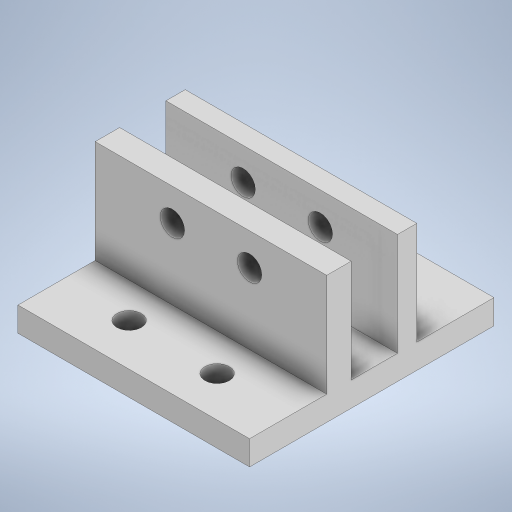
# Autodesk Inventor part: arm_to_tower_adapter
Saved by Autodesk Inventor 2024 (Build 280153000, 153)
## iProperties
Created: 2023-11-02
Part Number: arm_to_tower_adapter
Material: Generic
Document SubType Name: Modeling
Designer: dimademler
Density: 1 g/cm^3
Appearance: Default
Author: dimademler
Autodesk Inventor part; units mm, degrees
ref_plane "YZ Plane" through (0, 0, 0) normal (1, 0, 0) x (0, 1, 0)
ref_plane "XZ Plane" through (0, 0, 0) normal (0, 1, 0) x (-1, 0, 0)
ref_plane "XY Plane" through (0, 0, 0) normal (0, 0, 1) x (1, 0, 0)
sketch "Sketch1" plane through (0, 0, 0) normal (0, 0, 1) x (1, 0, 0)
  line L0 (0, 0) -> (-45.72, 0)
  line L1 (-45.72, 0) -> (-45.72, 20.32)
  line L2 (-45.72, 20.32) -> (0, 20.32)
  line L3 (0, 20.32) -> (0, 0)
  dimension "d0" = 45.72
  dimension "d1" = 20.32
  constraints: 8 end point, 2 parallel, 1 horizontal, 1 perpendicular
  measures "d0" distance of L0.start L0.end
  measures "d1" distance of L0.end L1.end
extrude "Extrusion1" add sketch "Sketch1" along normal blind 4.826
sketch "Sketch2" plane through (-45.72, 0, 0) normal (0, -1, 0) x (1, 0, 0)
  line L0 (45.72, 0) -> (45.72, 4.826) projected
  line L1 (0, 0) -> (0, 4.826) projected
  line L2 (0, 0) -> (45.72, 0) projected
  line L3 (0, 4.826) -> (45.72, 4.826) projected
  line L4 (45.72, 0) -> (45.72, -28.194)
  line L5 (45.72, 4.826) -> (45.72, 20.066)
  line L6 (45.72, 20.066) -> (0, 20.066)
  line L7 (0, 20.066) -> (0, 4.826)
  line L8 (0, 0) -> (0, -28.194)
  line L9 (0, -28.194) -> (45.72, -28.194)
  line L10 (45.72, 0) -> (45.72, 4.826)
  line L11 (0, 4.826) -> (0, 0)
  dimension "d4" = 28.194
  dimension "d5" = 15.24
  constraints: 16 end point, 4 vertical, 3 perpendicular, 1 point on line
  measures "d4" distance of L0.start L4.end
  measures "d5" distance of L0.end L5.end
extrude "Extrusion2" add sketch "Sketch2" along normal blind 4.826
sketch "Sketch3" plane through (-45.72, 0, 0) normal (0, 1, 0) x (1, 0, 0)
  line L0 (45.72, 0) -> (0, 0) projected
  line L1 (45.72, 28.194) -> (45.72, 0) projected
  line L2 (0, 28.194) -> (45.72, 28.194) projected
  line L3 (0, 0) -> (0, 28.194) projected
  line L4 (22.86, 0) -> (22.86, 9.144) construction
  line L5 (22.86, 9.144) -> (45.72, 9.144)
  line L6 (22.86, 9.144) -> (0, 9.144)
  line L7 (45.72, 9.144) -> (45.72, 12.954)
  line L8 (45.72, 28.194) -> (45.72, -20.066) projected
  line L9 (45.72, 12.954) -> (0, 12.954)
  line L10 (0, 12.954) -> (0, 9.144)
  dimension "d8" = 9.144
  dimension "d9" = 3.81
  constraints: 12 end point, 5 point on line, 2 perpendicular, 1 collinear, 1 midpoint, 1 vertical
  measures "d8" distance of L4.start L4.end
  measures "d9" distance of L5.end L7.end
extrude "Extrusion3" add sketch "Sketch3" along normal blind 20.32 contours L5 L6 L3 L9 L1
sketch "Sketch4" plane through (0, 0, -12.954) normal (0, 0, -1) x (-1, 0, 0)
  line L0 (0, 0) -> (0, 20.32) projected
  line L1 (0, 20.32) -> (45.72, 20.32) projected
  line L2 (45.72, 0) -> (45.72, 20.32) projected
  line L3 (45.72, 0) -> (0, 0) projected
  line L4 (22.86, 20.32) -> (22.86, 13.97) construction
  line L5 (22.86, 13.97) -> (30.48, 13.97) construction
  circle A0 centre (30.48, 13.97) radius 2.413
  circle A1 centre (15.24, 13.97) radius 2.413
  dimension "d12" = 6.35
  dimension "d13" = 7.62
  dimension "d14" = 4.826
  constraints: 4 end point, 2 centre point, 1 coincident, 1 horizontal, 1 midpoint, 1 symmetric about line, 1 vertical, 1 other
  measures "d12" distance of L4.start L4.end
  measures "d13" distance of L4.end L5.end
  measures "d14" diameter of A0
extrude "Extrusion4" cut sketch "Sketch4" against normal through all contours A0 | A1
sketch "Sketch5" plane through (-45.72, 0, 0) normal (0, 1, 0) x (1, 0, 0)
  line L0 (45.72, 12.954) -> (0, 12.954) projected
  line L1 (0, 28.194) -> (45.72, 28.194) projected
  line L2 (45.72, 28.194) -> (45.72, 12.954) construction
  line L3 (0, 12.954) -> (0, 28.194) projected
  line L4 (45.72, 28.194) -> (45.72, -20.066) projected
  line L5 (45.72, 28.194) -> (45.72, 12.954) construction
  line L6 (45.72, 20.574) -> (0, 20.574) construction
  line L7 (22.86, 12.954) -> (22.86, 20.574) construction
  line L8 (22.86, 20.574) -> (13.97, 20.574) construction
  line L9 (22.86, 20.574) -> (31.75, 20.574) construction
  circle A0 centre (31.75, 20.574) radius 2.413
  circle A1 centre (13.97, 20.574) radius 2.413
  line L10 (45.72, 4.064) -> (0, 4.572) construction
  line L11 (0, 0) -> (0, 9.144) projected
  circle A2 centre (31.3866, -12.1315) radius 2.413
  circle A3 centre (13.611, -11.7365) radius 2.413
  point P0 (45.72, 0)
  dimension "d17" = 8.89
  dimension "d18" = 8.89
  dimension "d19" = 4.826
  dimension "d20" = 4.826
  constraints: 12 end point, 6 midpoint, 4 centre point, 2 coincident, 2 point on line, 2 symmetric about line, 1 collinear, 1 horizontal, 1 perpendicular, 2 other
  measures "d17" distance of L7.end L8.end
  measures "d18" distance of L7.end L9.end
  measures "d19" diameter of A0
  measures "d20" diameter of A1
extrude "Extrusion5" cut sketch "Sketch5" against normal through all contours A0 | A1 | A2 | A3
body "Solid1"
